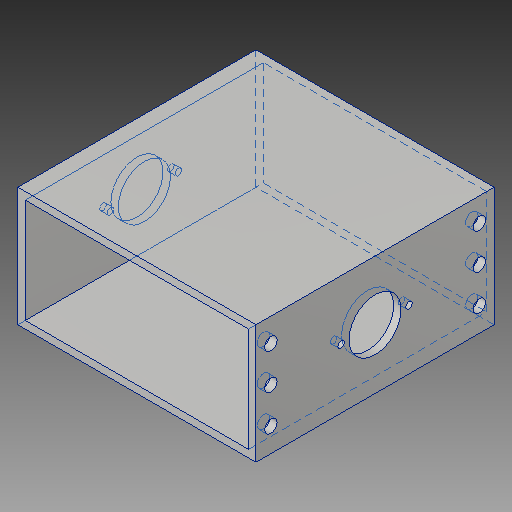
# Autodesk Inventor part: Arm 4 inch
Saved by Autodesk Inventor 2019 (Build 230136000, 136)
## iProperties
Created: 2018-09-22
Part Number: Arm 4 inch
Material: Aluminum 6061
Document SubType Name: Modeling
Designer: Adhik
Density: 2.7 g/cm^3
Appearance: Aluminum - Flat
Mass: 246.398 g
Surface Area: 602.146 cm^2
Volume: 91.2586 cm^3
Author: Adhik
Autodesk Inventor part; units mm, degrees
ref_plane "YZ Plane" through (0, 0, 0) normal (1, 0, 0) x (0, 1, 0)
ref_plane "XZ Plane" through (0, 0, 0) normal (0, 1, 0) x (-1, 0, 0)
ref_plane "XY Plane" through (0, 0, 0) normal (0, 0, 1) x (1, 0, 0)
sketch "Sketch1" plane through (0, 0, 0) normal (0, 0, 1) x (1, 0, 0)
  line L0 (-71.12, 0) -> (71.12, 0) construction
  line L1 (0, -35.56) -> (0, 35.56) construction
  line L2 (-50.8, 25.4) -> (50.8, 25.4)
  line L3 (50.8, 25.4) -> (50.8, -25.4)
  line L4 (50.8, -25.4) -> (-50.8, -25.4)
  line L5 (-50.8, -25.4) -> (-50.8, 25.4)
  line L6 (-47.625, 22.225) -> (47.625, 22.225)
  line L7 (47.625, 22.225) -> (47.625, -22.225)
  line L8 (47.625, -22.225) -> (-47.625, -22.225)
  line L9 (-47.625, -22.225) -> (-47.625, 22.225)
  point P0 (0, 0)
  point P1 (-50.8, 0)
  point P2 (0, 25.4)
  point P3 (-47.625, 0)
  point P4 (0, 22.225)
  dimension "d0" = 50.8
  dimension "d1" = 3.175
  dimension "d11" = 101.6
  dimension "d12" = 3.175
  constraints: 16 end point, 4 midpoint, 4 parallel, 4 point on line, 2 horizontal, 2 perpendicular
  measures "d0" distance of L4.end L2.start
  measures "d1" distance between parallel lines of L2 L6
  measures "d11" distance of L2.start L2.end
  measures "d12" distance between parallel lines of L5 L9
extrude "Extrusion1" add sketch "Sketch1" along normal mid plane 101.6
sketch "Sketch2" plane through (50.8, -25.4, 50.8) normal (1, 0, 0) x (0, 0, -1)
  line L0 (121.92, 25.4) -> (-20.32, 25.4) construction
  line L1 (50.8, -10.16) -> (50.8, 60.96) construction
  line L2 (6.35, 40.64) -> (95.25, 40.64) construction
  line L3 (95.25, 40.64) -> (95.25, 10.16) construction
  line L4 (95.25, 10.16) -> (6.35, 10.16) construction
  line L5 (6.35, 10.16) -> (6.35, 40.64) construction
  circle A0 centre (6.35, 40.64) radius 2.667
  circle A1 centre (95.25, 40.64) radius 2.667
  circle A2 centre (95.25, 10.16) radius 2.667
  circle A3 centre (6.35, 10.16) radius 2.667
  line L6 (0, 0) -> (0, 50.8) construction
  circle A4 centre (6.35, 25.4) radius 2.667
  circle A5 centre (95.25, 25.4) radius 2.667
  point P0 (50.8, 25.4)
  point P1 (50.8, 40.64)
  dimension "d4" = 5.334
  dimension "d5" = 6.35
  dimension "d6" = 15.24
  constraints: 8 end point, 6 centre point, 5 coincident, 5 equal radius, 3 midpoint, 2 parallel, 2 point on line, 1 horizontal, 1 perpendicular
  measures "d4" diameter of A0
  measures "d5" distance between parallel lines of L6 L5
  measures "d6" distance between parallel lines of L2 L0
extrude "Extrusion3" cut sketch "Sketch2" against normal up to next
sketch "Sketch3" plane through (-50.8, -25.4, 50.8) normal (-1, 0, 0) x (0, 0, 1)
  circle A0 centre (-50.8, 25.4) radius 11.1125
  dimension "d13" = 22.225
  constraints: 1 centre point, 1 coincident
  measures "d13" diameter of A0
extrude "Extrusion4" cut sketch "Sketch3" against normal through all
sketch "Sketch4" plane through (-50.8, -25.4, 50.8) normal (-1, 0, 0) x (0, 0, 1)
  line L0 (-121.92, 25.4) -> (20.32, 25.4) construction
  line L1 (-50.8, -10.16) -> (-50.8, 60.96) construction
  circle A0 centre (-50.8, 25.4) radius 12.7 construction
  circle A1 centre (-65.278, 25.4) radius 1.778 construction
  circle A2 centre (-65.278, 25.4) radius 1.397
  circle A3 centre (-36.322, 25.4) radius 1.397
  dimension "d16" = 25.4
  dimension "d17" = 3.556
  dimension "d18" = 2.794
  constraints: 4 centre point, 2 coincident, 1 point on line, 1 symmetric about line, 1 tangent, 1 other
  measures "d16" diameter of A0
  measures "d17" diameter of A1
  measures "d18" diameter of A2
extrude "Extrusion5" cut sketch "Sketch4" against normal through all
equation "\"d12\" = d1"
body "Solid1"
